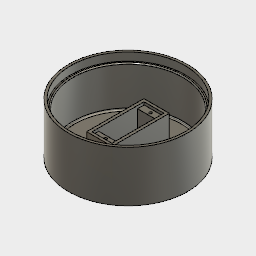
intelligent light (Autodesk Fusion 360 design; units mm, degrees)
Autodesk Fusion 360 part; units mm, degrees
note: some values were not read from the file. Set by a fixed rule: which sketch regions a step uses.
sketch "Sketch1" plane through (0, 0, 0) normal (0, 1, 0) x (1, 0, 0) in component "Emax Servo"
  line L0 (-12, -9.5) -> (8, -9.5)
  line L1 (8, -9.5) -> (12, -7.5)
  line L2 (12, -7.5) -> (12, 5.8)
  line L3 (12, 5.8) -> (16.1, 5.8)
  line L4 (16.1, 5.8) -> (16.1, 7.5)
  line L5 (16.1, 7.5) -> (12, 7.5)
  line L6 (12, 7.5) -> (12, 11.5)
  line L7 (12, 11.5) -> (-12, 11.5)
  line L8 (-12, 11.5) -> (-12, 7.5)
  line L9 (-12, 7.5) -> (-16.1, 7.5)
  line L10 (-16.1, 7.5) -> (-16.1, 5.8)
  line L11 (-16.1, 5.8) -> (-12, 5.8)
  line L12 (-12, 5.8) -> (-12, -9.5)
  dimension "d2" = 24
  dimension "d3" = 20
  dimension "d4" = 4.1
  dimension "d5" = 4
  dimension "d6" = 15.3
  dimension "d7" = 1.7
  dimension "d8" = 12
  dimension "d9" = 11.5
  measures "d2" distance of L6.end L7.end
  measures "d3" distance of L0.start L0.end
  measures "d4" distance of L4.end L5.end
  measures "d5" distance of L7.end L8.end
  measures "d6" distance of L0.start L11.end
  measures "d7" distance of L9.end L10.end
  measures "d8" distance of origin L12
  measures "d9" distance of origin L7
extrude "Extrude1" add sketch "Sketch1" along normal blind 12 makes body 1 in component "Emax Servo"
sketch "Sketch2" plane through (0, 0, -7.5) normal (0, 0, -1) x (-1, 0, 0) in component "Emax Servo"
  line L0 (-16.1, 0) -> (-12, 0)
  line L1 (-12, 0) -> (-12, 12)
  line L2 (-12, 12) -> (-16.1, 12)
  line L3 (-16.1, 12) -> (-16.1, 0)
  circle A0 centre (-14.15, 6) radius 0.95
  line L4 (-14.15, 6) -> (-14.1645, 12) construction
  line L5 (-14.15, 6) -> (-14.1645, 0) construction
  line L6 (-12, 0) -> (12, 0)
  line L7 (0, 15) -> (0, -5) construction
  circle A1 centre (14.15, 6) radius 0.95
  line L8 (14.15, 6) -> (14.1645, 12) construction
  line L9 (14.15, 6) -> (14.1645, 0) construction
  dimension "d12" = 1.9
  dimension "d14" = 1.95
  measures "d12" diameter of A0
  measures "d14" distance of L3 A0.centre
extrude "Extrude2" cut sketch "Sketch2" against normal through all contours A0 | A1 bodies 1 in component "Emax Servo"
sketch "Sketch3" plane through (0, 0, -11.5) normal (0, 0, -1) x (-1, 0, 0) in component "Emax Servo"
  line L0 (-12, 0) -> (12, 0)
  line L1 (12, 0) -> (12, 12)
  line L2 (12, 12) -> (-12, 12)
  line L3 (-12, 12) -> (-12, 0)
  circle A0 centre (-6.25, 6) radius 5.75
  line L4 (12, 6) -> (-12, 6) construction
  circle A1 centre (-0.5, 6) radius 3.125
  dimension "d17" = 11.5
  dimension "d18" = 6.25
  measures "d17" diameter of A0
  measures "d18" diameter of A1
extrude "Extrude3" add sketch "Sketch3" along normal blind 3.5 contours A0 A1 | A0 A1 | A0 A1 bodies 1 in component "Emax Servo"
sketch "Sketch4" plane through (0, 0, -15) normal (0, 0, -1) x (-1, 0, 0) in component "Emax Servo"
  arc A0 (-1.3492, 2.9926) -> (-1.3492, 9.0074) centre (-0.5, 6) ccw
  arc A1 (-1.3492, 9.0074) -> (-1.3492, 2.9926) centre (-6.25, 6) ccw
  circle A2 centre (-6.25, 6) radius 2.25
  dimension "d21" = 4.5
  measures "d21" diameter of A2
extrude "Extrude4" add sketch "Sketch4" along normal blind 4 contours A2 bodies 1 in component "Emax Servo"
sketch "Sketch5" plane through (0, 0, -15) normal (0, 0, -1) x (-1, 0, 0) in component "Emax Servo"
  circle A0 centre (-6.25, 6) radius 2.25
  arc A1 (-1.3492, 2.9926) -> (-1.3492, 9.0074) centre (-0.5, 6) ccw
  arc A2 (-1.3492, 9.0074) -> (-1.3492, 2.9926) centre (-6.25, 6) ccw
  circle A3 centre (0, 6) radius 1
  line L0 (-12, 6) -> (-12, 12)
  dimension "d24" = 2
  dimension "d25" = 12
  measures "d24" diameter of A3
  measures "d25" distance of A3.centre L0
extrude "Extrude5" add sketch "Sketch5" along normal blind 1 contours A3 bodies 1 in component "Emax Servo"
sketch "Sketch1 (2)" plane through (0, 0, 0) normal (0, 1, 0) x (1, 0, 0) in component "Servo Horn"
  circle A0 centre (0, 0) radius 3.5
  circle A1 centre (13.5, 0) radius 1.875
  line L0 (-0.0174, -3.5) -> (13.5, -1.875)
  line L1 (-5, 0) -> (18, 0)
  line L2 (-0.0174, 3.5) -> (13.5, 1.875)
  dimension "d28" = 7
  dimension "d29" = 3.75
  dimension "d30" = 13.5
  measures "d28" diameter of A0
  measures "d29" diameter of A1
  measures "d30" distance of A0.centre A1.centre
extrude "Extrude1'" add sketch "Sketch1 (2)" along normal blind 2 separate body contours A0 L1 L2 | A0 A1 L0 L1 | A0 L0 L1 | A0 A1 L1 L2 | A1 L1 | A1 L1 makes body 2 in component "Servo Horn"
sketch "Sketch2 (2)" plane through (0, 2, 0) normal (0, 1, 0) x (-1, 0, 0) in component "Servo Horn"
  arc A0 (0.0174, -3.5) -> (0.0174, 3.5) centre (0, 0) ccw
  line L0 (0.0174, 3.5) -> (-13.5, 1.875)
  arc A1 (-13.5, 1.875) -> (-13.5, -1.875) centre (-13.5, 0) ccw
  line L1 (-13.5, -1.875) -> (0.0174, -3.5)
  circle A2 centre (0, 0) radius 3.5
  dimension "d33" = 7
  measures "d33" diameter of A2
extrude "Extrude2'" add sketch "Sketch2 (2)" along normal blind 2.5 contours A0 L0 L1 A2 bodies 2 in component "Servo Horn"
sketch "Sketch3 (2)" plane through (0, 4.5, 0) normal (0, 1, 0) x (-1, 0, 0) in component "Servo Horn"
  arc A0 (0.0174, -3.5) -> (0.0174, 3.5) centre (0, 0) ccw
  line L0 (0.0174, 3.5) -> (-0.8464, 3.3961)
  arc A1 (-0.8464, 3.3961) -> (-0.8464, -3.3961) centre (0, 0) ccw
  line L1 (-0.8464, -3.3961) -> (0.0174, -3.5)
  circle A2 centre (0, 0) radius 2.25
  dimension "d36" = 4.5
  measures "d36" diameter of A2
extrude "Extrude3'" cut sketch "Sketch3 (2)" against normal up to surface (2.5 mm away) contours A2 bodies 2 in component "Servo Horn"
sketch "Sketch4 (2)" plane through (0, 0, 0) normal (1, 0, 0) x (0, 0, -1) in component "Servo Horn"
sketch "Sketch5 (2)" plane through (0, 2, 0) normal (0, 1, 0) x (-1, 0, 0) in component "Servo Horn"
  circle A0 centre (0, 0) radius 2.25
  circle A1 centre (0, 0) radius 1.2
  dimension "d39" = 2.4
  measures "d39" diameter of A1
extrude "Extrude4'" cut sketch "Sketch5 (2)" against normal through all contours A1 bodies 2 in component "Servo Horn"
sketch "Sketch6" plane through (0, 0, 0) normal (0, -1, 0) x (1, 0, 0) in component "Servo Horn"
  circle A0 centre (0, 0) radius 1.2
  arc A1 (-0.0174, 3.5) -> (-0.0174, -3.5) centre (0, 0) ccw
  line L0 (-0.0174, -3.5) -> (13.5, -1.875)
  arc A2 (13.5, -1.875) -> (13.5, 1.875) centre (13.5, 0) ccw
  line L1 (13.5, 1.875) -> (-0.0174, 3.5)
  circle A3 centre (0, 0) radius 2.375
  dimension "d41" = 4.75
  measures "d41" diameter of A3
extrude "Extrude5'" cut sketch "Sketch6" against normal blind 1 contours A3 bodies 2 in component "Servo Horn"
sketch "Sketch7" plane through (0, 2, 0) normal (0, 1, 0) x (-1, 0, 0) in component "Servo Horn"
  arc A0 (-0.8464, 3.3961) -> (-0.8464, -3.3961) centre (0, 0) ccw
  line L0 (-0.8464, 3.3961) -> (-13.5, 1.875)
  arc A1 (-13.5, 1.875) -> (-13.5, -1.875) centre (-13.5, 0) ccw
  line L1 (-13.5, -1.875) -> (-0.8464, -3.3961)
  circle A2 centre (-13.5, 0) radius 0.5
  circle A3 centre (-8, 0) radius 0.5
  circle A4 centre (-10.75, 0) radius 0.5
  dimension "d44" = 1
  dimension "d45" = 1
  dimension "d46" = 1
  dimension "d47" = 2.75
  dimension "d48" = 2.75
  measures "d44" diameter of A2
  measures "d45" diameter of A4
  measures "d46" diameter of A3
  measures "d47" distance of A1.centre A4.centre
  measures "d48" distance of A3.centre A4.centre
extrude "Extrude6" cut sketch "Sketch7" against normal through all contours A2 | A3 | A4 bodies 2 in component "Servo Horn"
sketch "Sketch8" plane through (0, 0, 0) normal (0, 1, 0) x (1, 0, 0) in component "Servo Horn"
sketch "Sketch1 (3)" plane through (0, 0, 0) normal (0, 1, 0) x (1, 0, 0) in component "Base"
  circle A0 centre (0, 0) radius 37.5
  dimension "d50" = 75
  measures "d50" diameter of A0
extrude "Extrude1''" add sketch "Sketch1 (3)" along normal blind 32 separate body makes body 3 in component "Base"
sketch "Sketch2 (3)" plane through (0, 32, 0) normal (0, 1, 0) x (-1, 0, 0) in component "Base"
  circle A0 centre (0, 0) radius 37.5
  circle A1 centre (0, 0) radius 36
  dimension "d53" = 1.5
  measures "d53" distance of A0 A1
extrude "Extrude2''" cut sketch "Sketch2 (3)" against normal blind 5 contours A1 bodies 3 in component "Base"
sketch "Sketch3 (3)" plane through (0, 27, 0) normal (0, 1, 0) x (-1, 0, 0) in component "Base"
  circle A0 centre (0, 0) radius 36
  circle A1 centre (0, 0) radius 34.5
  circle A2 centre (0, 0) radius 37.5
  dimension "d56" = 3
  measures "d56" distance of A1 A2
extrude "Extrude3''" cut sketch "Sketch3 (3)" against normal up to surface (25.5 mm away) contours A1 bodies 3 in component "Base"
sketch "Sketch4 (3)" plane through (0, 1.5, 0) normal (0, 1, 0) x (-1, 0, 0) in component "Base"
  circle A0 centre (0, 0) radius 34.5
  line L0 (-8, 18) -> (8, 18)
  line L1 (8, 18) -> (8, -18)
  line L2 (8, -18) -> (-8, -18)
  line L3 (-8, -18) -> (-8, 18)
  line L4 (-8, 18) -> (8, -18) construction
  line L5 (8, 18) -> (-8, -18) construction
  dimension "d59" = 16
  dimension "d60" = 36
  measures "d59" distance of L1.end L2.end
  measures "d60" distance of L0.end L1.end
extrude "Extrude4''" add sketch "Sketch4 (3)" along normal blind 17.5 contours L0 L1 L2 L3 bodies 3 in component "Base"
sketch "Sketch5 (3)" plane through (0, 19, 0) normal (0, 1, 0) x (-1, 0, 0) in component "Base"
  line L0 (-8, -18) -> (8, -18)
  line L1 (8, -18) -> (8, 18)
  line L2 (8, 18) -> (-8, 18)
  line L3 (-8, 18) -> (-8, -18)
  line L4 (-6.25, 12.25) -> (6.25, 12.25)
  line L5 (6.25, 12.25) -> (6.25, -12.25)
  line L6 (6.25, -12.25) -> (-6.25, -12.25)
  line L7 (-6.25, -12.25) -> (-6.25, 12.25)
  line L8 (-6.25, 12.25) -> (6.25, -12.25) construction
  line L9 (6.25, 12.25) -> (-6.25, -12.25) construction
  dimension "d63" = 24.5
  dimension "d64" = 12.5
  measures "d63" distance of L4.start L6.end
  measures "d64" distance of L5.end L6.end
extrude "Extrude5''" cut sketch "Sketch5 (3)" against normal up to surface (17.5 mm away) contours L4 L5 L6 L7 bodies 3 in component "Base"
sketch "Sketch6 (2)" plane through (0, 0, 18) normal (0, 0, 1) x (1, 0, 0) in component "Base"
  line L0 (-8, 1.5) -> (8, 1.5)
  line L1 (8, 1.5) -> (8, 19)
  line L2 (8, 19) -> (-8, 19)
  line L3 (-8, 19) -> (-8, 1.5)
sketch "Sketch7 (2)" plane through (0, 0, 18) normal (0, 0, 1) x (1, 0, 0) in component "Base"
  line L0 (-5, 1.5) -> (5, 1.5)
  line L1 (5, 1.5) -> (5, 11.5)
  line L2 (5, 11.5) -> (-5, 11.5)
  line L3 (-5, 11.5) -> (-5, 1.5)
  line L4 (-8, 1.5) -> (8, 1.5)
  line L5 (-6.25, 1.5) -> (6.25, 1.5)
  line L6 (8, 1.5) -> (8, 19)
  line L7 (-8, 19) -> (-8, 1.5)
  dimension "d68" = 10
  dimension "d69" = 3
  dimension "d70" = 3
  measures "d68" distance of L0.end L1.end
  measures "d69" distance of L1 L6
  measures "d70" distance of L3 L7
extrude "Extrude6'" cut sketch "Sketch7 (2)" against normal up to surface (5.75 mm away) bodies 3 in component "Base"
sketch "Sketch8 (2)" plane through (0, 19, 0) normal (0, 1, 0) x (-1, 0, 0) in component "Base"
  line L0 (6.25, -12.25) -> (-6.25, -12.25)
  line L1 (-6.25, -12.25) -> (-6.25, 12.25)
  line L2 (-6.25, 12.25) -> (6.25, 12.25)
  line L3 (6.25, 12.25) -> (6.25, -12.25)
  line L4 (-8, -18) -> (8, -18)
  line L5 (8, -18) -> (8, 18)
  line L6 (8, 18) -> (-8, 18)
  line L7 (-8, 18) -> (-8, -18)
  circle A0 centre (0, -14.15) radius 0.85
  circle A1 centre (0, 14.15) radius 0.85
  dimension "d73" = 1.7
  dimension "d74" = 14.15
  dimension "d75" = 1.7
  dimension "d76" = 14.15
  measures "d73" diameter of A0
  measures "d74" distance of origin A0.centre
  measures "d75" diameter of A1
  measures "d76" distance of origin A1.centre
extrude "Extrude7" cut sketch "Sketch8 (2)" against normal blind 10 contours A0 | A1 bodies 3 in component "Base"
sketch "Sketch9" plane through (0, 19, 0) normal (0, 1, 0) x (-1, 0, 0) in component "Base"
  circle A0 centre (0, 14.15) radius 0.85
  circle A1 centre (0, -14.15) radius 0.85
  line L0 (6.25, -12.25) -> (-6.25, -12.25)
  line L1 (-6.25, -12.25) -> (-6.25, 12.25)
  line L2 (-6.25, 12.25) -> (6.25, 12.25)
  line L3 (6.25, 12.25) -> (6.25, -12.25)
  line L4 (-8, -18) -> (8, -18)
  line L5 (8, -18) -> (8, 18)
  line L6 (8, 18) -> (-8, 18)
  line L7 (-8, 18) -> (-8, -18)
  line L8 (-6.25, 16.375) -> (6.25, 16.375)
  line L9 (6.25, 16.375) -> (6.25, -16.375)
  line L10 (6.25, -16.375) -> (-6.25, -16.375)
  line L11 (-6.25, -16.375) -> (-6.25, 16.375)
  line L12 (-6.25, 16.375) -> (6.25, -16.375) construction
  line L13 (6.25, 16.375) -> (-6.25, -16.375) construction
  dimension "d79" = 32.75
  dimension "d80" = 12.5
  measures "d79" distance of L8.end L9.end
  measures "d80" distance of L9.end L10.end
extrude "Extrude8" cut sketch "Sketch9" against normal blind 1.75 contours L0 L9 L10 L11 | L0 L1 L2 L3 L9 L11 | L2 L8 L9 L11 bodies 3 in component "Base"
fillet "Fillet1" radius 1 6 edges at (6.5, 1.5, 18) (-6.5, 1.5, 18) (-8, 1.5, 0) (32.1653, 1.5, -12.4757) (0, 1.5, -18) (8, 1.5, 0) on bodies 3 in component "Base"
fillet "Fillet2" radius 0.65 1 edges at (32.1653, 27, 12.4757) on bodies 3 in component "Base"
component "Emax Servo" placed x (1, 0, 0) y (0, 1, 0) z (0, 0, 1) at (0, 0, 0)
component "Servo Horn" placed x (1, 0, 0) y (0, 1, 0) z (0, 0, 1) at (0, 0, 0)
component "Base" placed x (1, 0, 0) y (0, 1, 0) z (0, 0, 1) at (0, 0, 0)
